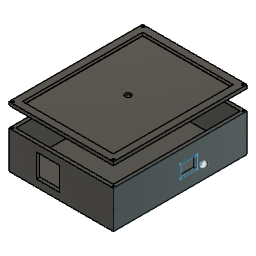
FireAlarmTx v3 (Autodesk Fusion 360 design; units mm, degrees)
Autodesk Fusion 360 part; units mm, degrees
sketch "Boceto47" plane through (0, 0, 0) normal (0, 1, 0) x (1, 0, 0)
  line L0 (0, 0) -> (107, 0)
  line L1 (107, 0) -> (107, 137)
  line L2 (107, 137) -> (0, 137)
  line L3 (0, 137) -> (0, 0)
  line L4 (3.5, 3.5) -> (103.5, 3.5)
  line L5 (103.5, 3.5) -> (103.5, 133.5)
  line L6 (103.5, 133.5) -> (3.5, 133.5)
  line L7 (3.5, 133.5) -> (3.5, 3.5)
  dimension "d114" = 107
  dimension "d115" = 137
  dimension "d117" = 4.9497
  dimension "d118" = 100
  dimension "d119" = 130
  constraint horizontal L0
  constraint vertical L1
  constraint horizontal L2
  constraint vertical L3
  constraint coincident L0.start L3.end
  constraint horizontal L4
  constraint vertical L5
  constraint horizontal L6
  constraint vertical L7
  measures "d114" distance of L0.start L0.end
  measures "d115" distance of L0.start L2.end
  measures "d117" distance of L0.start L4.start
  measures "d118" distance of L4.start L4.end
  measures "d119" distance of L4.start L6.end
sketch "Boceto49" plane through (0, 0, 0) normal (0, 1, 0) x (1, 0, 0)
  line L0 (0, 0) -> (107, 0)
  line L1 (107, 0) -> (107, 137)
  line L2 (107, 137) -> (0, 137)
  line L3 (0, 137) -> (0, 0)
  circle A0 centre (1.75, 1.75) radius 1.1
  circle A1 centre (105.25, 1.75) radius 1.1
  circle A2 centre (105.25, 135.25) radius 1.1
  circle A3 centre (1.75, 135.25) radius 1.1
  line L4 (8.5, 128.4999) -> (98.5, 128.4999)
  line L5 (98.5, 128.4999) -> (98.5, 8.4999)
  line L6 (98.5, 8.4999) -> (8.5, 8.4999)
  line L7 (8.5, 8.4999) -> (8.5, 128.4999)
  circle A4 centre (53.5, 68.4999) radius 3
  dimension "d120" = 107
  dimension "d121" = 137
  dimension "d123" = 2.4749
  dimension "d124" = 2.2
  dimension "d126" = 2.4749
  dimension "d127" = 2.2
  dimension "d129" = 2.4749
  dimension "d130" = 2.2
  dimension "d132" = 2.4749
  dimension "d133" = 2.2
  dimension "d149" = 90
  dimension "d150" = 120
  dimension "d162" = 6
  constraint horizontal L0
  constraint vertical L1
  constraint horizontal L2
  constraint vertical L3
  constraint coincident L0.start L3.end
  constraint horizontal L4
  constraint vertical L5
  constraint horizontal L6
  constraint vertical L7
  measures "d120" distance of L0.start L0.end
  measures "d121" distance of L0.start L2.end
  measures "d123" distance of L0.start A0.centre
  measures "d124" diameter of A0
  measures "d126" distance of L0.end A1.centre
  measures "d127" diameter of A1
  measures "d129" distance of L1.end A2.centre
  measures "d130" diameter of A2
  measures "d132" distance of L2.end A3.centre
  measures "d133" diameter of A3
  measures "d149" distance of L4.start L4.end
  measures "d150" distance of L4.start L6.end
  measures "d162" diameter of A4
extrude "Extruir19" add sketch "Boceto47" against normal blind 3.5 contours L0 L1 L2 L3 | L4 L5 L6 L7 makes body 1
extrude "Extruir20" add sketch "Boceto47" along normal blind 35 bodies 1
move_body "Desplazar4" bodies 1 to x (1, 0, 0) y (0, 1, 0) z (0, 0, 1) at (0, -35, 0)
extrude "Extruir21" cut sketch "Boceto49" against normal blind 19 contours A0 | A1 | A2 | A3 bodies 1
sketch "Boceto50" plane through (0, 0, 0) normal (0, 1, 0) x (1, 0, 0)
  line L0 (3.9578, 10.1379) -> (88.9578, 10.1379)
  line L1 (88.9578, 10.1379) -> (88.9578, 102.1379)
  line L2 (88.9578, 102.1379) -> (3.9578, 102.1379)
  line L3 (3.9578, 102.1379) -> (3.9578, 10.1379)
  line L4 (103.0109, 38.2575) -> (89.0109, 38.2575)
  line L5 (89.0109, 38.2575) -> (89.0109, 20.2575)
  line L6 (89.0109, 20.2575) -> (103.0109, 20.2575)
  line L7 (103.0109, 20.2575) -> (103.0109, 38.2575)
  dimension "d140" = 85
  dimension "d141" = 92
  dimension "d142" = 14
  dimension "d143" = 18
  constraint horizontal L0
  constraint vertical L1
  constraint horizontal L2
  constraint vertical L3
  constraint horizontal L4
  constraint vertical L5
  constraint horizontal L6
  constraint vertical L7
  measures "d140" distance of L0.start L0.end
  measures "d141" distance of L0.start L2.end
  measures "d142" distance of L4.start L4.end
  measures "d143" distance of L4.start L6.end
extrude "Extruir22" add sketch "Boceto49" along normal blind 3.5 separate body contours L0 L1 L2 L3 | L4 L5 L6 L7 | A4 makes body 2
move_body "Desplazar5" bodies 1 to x (1, 0, 0) y (0, 1, 0) z (0, 0, 1) at (0, -3.5, 0)
move_body "Desplazar6" bodies 2 to x (1, 0, 0) y (0, 1, 0) z (0, 0, 1) at (0, -3.5, 0)
extrude "Extruir23" cut sketch "Boceto49" against normal blind 1.75 contours L4 L5 L6 L7 | A4 bodies 2
chamfer "Chaflán1" distance 0.5 angle 45 1 edges at (0.7244, 0, -135.6478) on bodies 2
chamfer "Chaflán2" distance 0.5 angle 45 1 edges at (104.2244, 0, -135.6478) on bodies 2
chamfer "Chaflán3" distance 0.5 angle 45 1 edges at (104.2244, 0, -2.1478) on bodies 2
chamfer "Chaflán4" distance 0.5 angle 45 1 edges at (0.7244, 0, -2.1478) on bodies 2
chamfer "Chaflán5" distance 1.5 angle 45 4 edges at (8.5, 0, -68.4999) (53.5, 0, -8.4999) (98.5, 0, -68.4999) (53.5, 0, -128.4999) on bodies 2
extrude "Extruir24" cut sketch "Boceto49" against normal blind 5 contours A4 bodies 2
move_body "Desplazar7" bodies 2 to x (1, 0, 0) y (0, 1, 0) z (0, 0, 1) at (0, 20, 0)
sketch "Boceto51" plane through (0, 0, 0) normal (0, 0, 1) x (1, 0, 0)
  line L0 (0, -3.5) -> (0, -42)
  line L1 (0, -42) -> (107, -42)
  line L2 (107, -42) -> (107, -3.5)
  line L3 (107, -3.5) -> (0, -3.5)
  line L4 (28.0002, -10.7505) -> (52.0002, -10.7505)
  line L5 (52.0002, -10.7505) -> (52.0002, -34.7505)
  line L6 (52.0002, -34.7505) -> (28.0002, -34.7505)
  line L7 (28.0002, -34.7505) -> (28.0002, -10.7505)
  dimension "d167" = 24
  dimension "d168" = 24
  constraint horizontal L4
  constraint vertical L5
  constraint horizontal L6
  constraint vertical L7
  measures "d167" distance of L4.start L4.end
  measures "d168" distance of L4.start L6.end
extrude "Extruir25" cut sketch "Boceto51" against normal blind 4 contours L4 L5 L6 L7 bodies 1
sketch "Boceto52" plane through (107, 0, 0) normal (1, 0, 0) x (0, 0, -1)
  line L0 (0, -3.5) -> (0, -42)
  line L1 (0, -42) -> (137, -42)
  line L2 (137, -42) -> (137, -3.5)
  line L3 (137, -3.5) -> (0, -3.5)
  line L4 (68.4993, -16.2507) -> (85.4993, -16.2507)
  line L5 (85.4993, -16.2507) -> (85.4993, -29.2507)
  line L6 (85.4993, -29.2507) -> (68.4993, -29.2507)
  line L7 (68.4993, -29.2507) -> (68.4993, -16.2507)
  circle A0 centre (91.4993, -27.7507) radius 1.6
  dimension "d172" = 17
  dimension "d173" = 13
  dimension "d178" = 3.2
  constraint horizontal L4
  constraint vertical L5
  constraint horizontal L6
  constraint vertical L7
  measures "d172" distance of L4.start L4.end
  measures "d173" distance of L4.start L6.end
  measures "d178" diameter of A0
extrude "Extruir26" cut sketch "Boceto52" against normal blind 4 contours L4 L5 L6 L7 bodies 1
extrude "Extruir27" cut sketch "Boceto52" against normal blind 3.5 contours A0 bodies 1
equation "d114 = 100 mm + ( 3.5 * 2 ) * 1 mm"
equation "d115 = 130 mm + ( 3.5 * 2 ) * 1 mm"
equation "d117 = ( ( 3.5 ^ 2 + 3.5 ^ 2 ) ^ ( 1 / 2 ) ) * 1 mm"
equation "d120 = 100 mm + ( 3.5 * 2 ) * 1 mm"
equation "d121 = 130 mm + ( 3.5 * 2 ) * 1 mm"
equation "d123 = ( ( ( 3.5 ^ 2 + 3.5 ^ 2 ) ^ ( 1 / 2 ) ) ) / 2 * 1 mm"
equation "d126 = ( ( ( 3.5 ^ 2 + 3.5 ^ 2 ) ^ ( 1 / 2 ) ) ) / 2 * 1 mm"
equation "d129 = ( ( ( 3.5 ^ 2 + 3.5 ^ 2 ) ^ ( 1 / 2 ) ) ) / 2 * 1 mm"
equation "d132 = ( ( ( 3.5 ^ 2 + 3.5 ^ 2 ) ^ ( 1 / 2 ) ) ) / 2 * 1 mm"
named bodies: "Box", "Cover"
